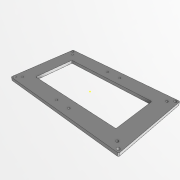
# Autodesk Inventor part: BoardMountingBracket
Saved by Autodesk Inventor 2018 (Build 220112000, 112)
## iProperties
Created: 2017-10-17
Part Number: BoardMountingBracket
Material: Generic
Document SubType Name: Modeling
Designer: jcj2131
Density: 1 g/cm^3
Appearance: Default
Author: jcj2131
Autodesk Inventor part; units mm, degrees
ref_plane "YZ Plane" through (0, 0, 0) normal (1, 0, 0) x (0, 1, 0)
ref_plane "XZ Plane" through (0, 0, 0) normal (0, 1, 0) x (-1, 0, 0)
ref_plane "XY Plane" through (0, 0, 0) normal (0, 0, 1) x (1, 0, 0)
sketch "Sketch1" plane through (0, 0, 0) normal (0, 1, 0) x (-1, 0, 0)
  line L0 (-120, 71.5) -> (120, 71.5)
  line L1 (120, 71.5) -> (120, 41.5)
  line L2 (120, 41.5) -> (-120, 41.5)
  line L3 (-120, 41.5) -> (-120, 71.5)
  line L4 (-120, -41.5) -> (120, -41.5)
  line L5 (120, -41.5) -> (120, -71.5)
  line L6 (120, -71.5) -> (-120, -71.5)
  line L7 (-120, -71.5) -> (-120, -41.5)
  line L8 (168, 0) -> (-168, 0) projected
  line L9 (0, -100.1) -> (0, 100.1) projected
  line L10 (120, 41.5) -> (-120, 41.5)
  line L11 (-120, 41.5) -> (-120, -41.5)
  line L12 (-120, -41.5) -> (120, -41.5)
  line L13 (120, -41.5) -> (120, 41.5)
  line L14 (90, 41.5) -> (-90, 41.5)
  line L15 (-90, 41.5) -> (-90, -41.5)
  line L16 (-90, -41.5) -> (90, -41.5)
  line L17 (90, -41.5) -> (90, 41.5)
  line L18 (-115, 66.5) -> (115, 66.5) construction
  line L19 (115, 66.5) -> (115, -66.5) construction
  line L20 (115, -66.5) -> (-115, -66.5) construction
  line L21 (-115, -66.5) -> (-115, 66.5) construction
  point P0 (0, 0)
  point P1 (0, 41.5)
  dimension "d0" = 240
  dimension "d2" = 30
  dimension "d4" = 143
  dimension "d55" = 30
  dimension "d56" = 5
  dimension "d57" = 5
  constraints: 40 end point, 10 parallel, 5 horizontal, 5 perpendicular, 2 equal length, 2 point on line, 1 collinear, 1 midpoint, 1 vertical alignment, 4 other
  measures "d0" distance of L0.start L0.end
  measures "d2" distance of L4.end L5.end
  measures "d4" distance between parallel lines of L6 L0
  measures "d55" distance between parallel lines of L17 L13
  measures "d56" distance between parallel lines of L0 L18
  measures "d57" distance between parallel lines of L1 L19
extrude "Extrusion1" add sketch "Sketch1" along normal blind 6.35 contours L0 L9 L2 L3 | L0 L1 L2 L9 | L2 L15 L8 L11 | L8 L15 L4 L11 | L13 L8 L17 L2 | L4 L9 L6 L7 | L13 L4 L17 L8 | L4 L5 L6 L9
sketch "Sketch2" plane through (0, 6.35, 0) normal (0, 1, 0) x (1, 0, 0)
  line L0 (-110, -61.5) -> (-10, -61.5)
  line L1 (-10, -61.5) -> (-10, 61.5)
  line L2 (-10, 61.5) -> (-110, 61.5)
  line L3 (-110, 61.5) -> (-110, -61.5)
  line L4 (-120, -71.5) -> (-120, 71.5) projected
  line L5 (-120, -71.5) -> (120, -71.5) projected
  line L6 (10, -61.5) -> (110, -61.5)
  line L7 (110, -61.5) -> (110, 61.5)
  line L8 (110, 61.5) -> (10, 61.5)
  line L9 (10, 61.5) -> (10, -61.5)
  circle A0 centre (-106, -57.5) radius 2.1
  circle A1 centre (-106, 57.5) radius 2.1
  circle A2 centre (-14, -57.5) radius 2.1
  circle A3 centre (-14, 57.5) radius 2.1
  circle A4 centre (14, -57.5) radius 2.1
  circle A5 centre (14, 57.5) radius 2.1
  circle A6 centre (106, -57.5) radius 2.1
  circle A7 centre (106, 57.5) radius 2.1
  point P0 (0, 0)
  point P1 (-120, -41.5)
  dimension "d7" = 123
  dimension "d8" = 100
  dimension "d9" = 10
  dimension "d10" = 10
  dimension "d11" = 100
  dimension "d12" = 123
  dimension "d13" = 20
  dimension "d14" = 4.2
  dimension "d15" = 4
  dimension "d16" = 4
  dimension "d17" = 4.2
  dimension "d18" = 4
  dimension "d19" = 4
  dimension "d20" = 4.2
  dimension "d21" = 4
  dimension "d22" = 4
  dimension "d23" = 4.2
  dimension "d24" = 4
  dimension "d25" = 4
  dimension "d26" = 4.2
  dimension "d27" = 4
  dimension "d28" = 4
  dimension "d29" = 4.2
  dimension "d30" = 4
  dimension "d31" = 4
  dimension "d32" = 4.2
  dimension "d33" = 4
  dimension "d34" = 4
  dimension "d35" = 4.2
  dimension "d36" = 4
  dimension "d37" = 4
  dimension "d38" = 10
  constraints: 16 end point, 8 centre point, 4 parallel, 2 horizontal, 2 perpendicular
  measures "d7" distance of L2.end L0.start
  measures "d8" distance of L0.start L0.end
  measures "d9" distance between parallel lines of L4 L3
  measures "d10" distance between parallel lines of L5 L0
  measures "d11" distance of L6.start L6.end
  measures "d12" distance of L6.end L7.end
  measures "d13" distance between parallel lines of L1 L9
  measures "d14" diameter of A0
  measures "d15" distance from line of L3 A0.centre
  measures "d16" distance from line of L0 A0.centre
  measures "d17" diameter of A1
  measures "d18" distance from line of L3 A1.centre
  measures "d19" distance from line of L2 A1.centre
  measures "d20" diameter of A2
  measures "d21" distance from line of L0 A2.centre
  measures "d22" distance from line of L1 A2.centre
  measures "d23" diameter of A3
  measures "d24" distance from line of L1 A3.centre
  measures "d25" distance from line of L2 A3.centre
  measures "d26" diameter of A4
  measures "d27" distance from line of L9 A4.centre
  measures "d28" distance from line of L6 A4.centre
  measures "d29" diameter of A5
  measures "d30" distance from line of L8 A5.centre
  measures "d31" distance from line of L9 A5.centre
  measures "d32" diameter of A6
  measures "d33" distance from line of L6 A6.centre
  measures "d34" distance from line of L7 A6.centre
  measures "d35" diameter of A7
  measures "d36" distance from line of L7 A7.centre
  measures "d37" distance from line of L8 A7.centre
  measures "d38" distance between parallel lines of L5 L6
extrude "Extrusion2" cut sketch "Sketch2" against normal through all contours A0 | A1 | A2 | A3 | A4 | A5 | A6 | A7
sketch "Sketch3" plane through (0, 6.35, 0) normal (0, 1, 0) x (1, 0, 0)
  circle A0 centre (-115, -66.5) radius 2.5
  line L0 (-120, -71.5) -> (-120, 71.5) projected
  line L1 (120, -71.5) -> (-120, -71.5) projected
  circle A1 centre (-115, 66.5) radius 2.5
  line L2 (-120, 41.5) -> (-120, 71.5) projected
  line L3 (-120, 71.5) -> (120, 71.5) projected
  circle A2 centre (115, -66.5) radius 2.5
  line L4 (120, -71.5) -> (120, 71.5) projected
  circle A3 centre (115, 66.5) radius 2.5
  line L5 (120, 41.5) -> (120, 71.5) projected
  point P0 (0, 0)
  point P1 (-120, -41.5)
  point P2 (120, -41.5)
  dimension "d41" = 5
  dimension "d42" = 5
  dimension "d43" = 5
  dimension "d44" = 5
  dimension "d45" = 5
  dimension "d46" = 5
  dimension "d47" = 5
  dimension "d48" = 5
  dimension "d49" = 5
  dimension "d50" = 5
  dimension "d51" = 5
  dimension "d52" = 5
  constraints: 4 centre point
  measures "d41" diameter of A0
  measures "d42" distance from line of L0 A0.centre
  measures "d43" distance from line of L1 A0.centre
  measures "d44" diameter of A1
  measures "d45" distance from line of L2 A1.centre
  measures "d46" distance from line of L3 A1.centre
  measures "d47" diameter of A2
  measures "d48" distance from line of L1 A2.centre
  measures "d49" distance from line of L4 A2.centre
  measures "d50" diameter of A3
  measures "d51" distance from line of L3 A3.centre
  measures "d52" distance from line of L5 A3.centre
extrude "Extrusion3" [suppressed]
hole "Hole1" at (115, 0, 66.5) at (115, 0, -66.5) at (-115, 0, -66.5) at (-115, 0, 66.5) direction (0, 1, 0) diameter 5.1 end through all
fillet "Fillet1" radius 2 8 edges at (90, 3.175, 41.5) (90, 3.175, -41.5) (-90, 3.175, 41.5) (-90, 3.175, -41.5) (-120, 3.175, 71.5) (-120, 3.175, -71.5) (120, 3.175, -71.5) (120, 3.175, 71.5)
sketch "Sketch5" plane through (0, 0, 0) normal (0, 1, 0) x (-1, 0, 0)
  point P0 (0, 0)
body "Solid1"
